Autodesk Fusion 360 part; units mm, degrees
note: some values were not read from the file. Set by a fixed rule: which face or edge a step refers to.
(part 2 of 2)
  line L1239 (389, 358.5) -> (389, 338.5)
  line L1240 (389, 338.5) -> (409, 338.5)
  line L1241 (409, 338.5) -> (409, 358.5)
  line L1242 (433, 358.5) -> (413, 358.5)
  line L1243 (413, 358.5) -> (413, 338.5)
  line L1244 (413, 338.5) -> (433, 338.5)
  line L1245 (433, 338.5) -> (433, 358.5)
  line L1246 (457, 358.5) -> (437, 358.5)
  line L1247 (437, 358.5) -> (437, 338.5)
  line L1248 (437, 338.5) -> (457, 338.5)
  line L1249 (457, 338.5) -> (457, 358.5)
  line L1250 (481, 358.5) -> (461, 358.5)
  line L1251 (461, 358.5) -> (461, 338.5)
  line L1252 (461, 338.5) -> (481, 338.5)
  line L1253 (481, 338.5) -> (481, 358.5)
  line L1254 (313, 382.5) -> (293, 382.5)
  line L1255 (293, 382.5) -> (293, 362.5)
  line L1256 (293, 362.5) -> (313, 362.5)
  line L1257 (313, 362.5) -> (313, 382.5)
  line L1258 (337, 382.5) -> (317, 382.5)
  line L1259 (317, 382.5) -> (317, 362.5)
  line L1260 (317, 362.5) -> (337, 362.5)
  line L1261 (337, 362.5) -> (337, 382.5)
  line L1262 (361, 382.5) -> (341, 382.5)
  line L1263 (341, 382.5) -> (341, 362.5)
  line L1264 (341, 362.5) -> (361, 362.5)
  line L1265 (361, 362.5) -> (361, 382.5)
  line L1266 (385, 382.5) -> (365, 382.5)
  line L1267 (365, 382.5) -> (365, 362.5)
  line L1268 (365, 362.5) -> (385, 362.5)
  line L1269 (385, 362.5) -> (385, 382.5)
  line L1270 (409, 382.5) -> (389, 382.5)
  line L1271 (389, 382.5) -> (389, 362.5)
  line L1272 (389, 362.5) -> (409, 362.5)
  line L1273 (409, 362.5) -> (409, 382.5)
  line L1274 (433, 382.5) -> (413, 382.5)
  line L1275 (413, 382.5) -> (413, 362.5)
  line L1276 (413, 362.5) -> (433, 362.5)
  line L1277 (433, 362.5) -> (433, 382.5)
  line L1278 (457, 382.5) -> (437, 382.5)
  line L1279 (437, 382.5) -> (437, 362.5)
  line L1280 (437, 362.5) -> (457, 362.5)
  line L1281 (457, 362.5) -> (457, 382.5)
  line L1282 (481, 382.5) -> (461, 382.5)
  line L1283 (461, 382.5) -> (461, 362.5)
  line L1284 (461, 362.5) -> (481, 362.5)
  line L1285 (481, 362.5) -> (481, 382.5)
  dimension "d46" = 486
  dimension "d47" = 385
  dimension "d50" = 5
  dimension "d51" = 2.5
  dimension "d52" = 20
  dimension "d53" = 20
  dimension "d56" = 24
  dimension "d57" = 24
  constraint horizontal L0
  constraint vertical L1
  constraint horizontal L2
  constraint vertical L3
  constraint coincident L0.start L3.end
  constraint coincident L3 L4.end
  constraint perpendicular L3 L4
  constraint coincident L0 L5.end
  constraint perpendicular L0 L5
  constraint horizontal L6
  constraint vertical L7
  constraint horizontal L8
  constraint vertical L9
  measures "d46" distance of L0.start L0.end
  measures "d47" distance of L0.start L2.end
  measures "d50" distance of L4.start L4.end
  measures "d51" distance of L4.start L5.end
  measures "d52" distance of L4.start L6.end
  measures "d53" distance of L4.start L8.end
extrude "Extrude2" add sketch "Sketch4" along normal blind 3 makes body 1
box "BoxPrimitive1" add length 24 width 22 height 51 placed x (0, 1, 0) y (-1, 0, 0) z (0, 0, 1) at (29, 369, 3) separate body makes body 2
extrude "Extrude3" cut 1 faces at (14.3333, 377, 3) along direction (0, 0, 1) blind 1 on bodies 2 bodies 2
extrude "Extrude4" cut 1 faces at (21.6667, 393, 20.6667) along direction (0, -1, 0) blind 2 on bodies 2 bodies 2
box "BoxPrimitive2" add length 19 width 19 height 4 placed x (0, 1, 0) y (1, 0, 0) z (0, 0, -1) at (8.5, 370.5, 4) bodies 2
shell "Shell1" thickness 2 removed faces 1 at (21.6667, 376.3333, 54) on bodies 2
copy_body "CopyPasteBodies1" bodies 2 makes body 3
move_body "Move1" bodies 3 to x (1, 0, 0) y (0, 1, 0) z (0, 0, 1) at (0, -24, 0)
copy_body "CopyPasteBodies2" bodies 3 2 makes body 4 makes body 5
move_body "Move2" bodies 4 5 to x (1, 0, 0) y (0, 1, 0) z (0, 0, 1) at (24, 0, 0)
copy_body "CopyPasteBodies3" bodies 3 2 4 5 makes body 6 makes body 7 makes body 8 makes body 9
move_body "Move3" bodies 6 7 8 9 to x (1, 0, 0) y (0, 1, 0) z (0, 0, 1) at (0, -72, 0)
box "BoxPrimitive3" add length 46 width 46 height -50 placed x (0, -1, 0) y (1, 0, 0) z (0, 0, 1) at (7, 319, 54) bodies 6 7 8 9
extrude "Extrude5" add 4 faces at (21.1667, 280.8333, 0) (38.8333, 280.8333, 0) (21.1667, 304.8333, 0) (38.8333, 304.8333, 0) along direction (0, 0, 1) blind 5 on bodies 6 bodies 6
shell "Shell2" thickness 2 removed faces 1 at (37.6667, 280.3333, 54) on bodies 6
extrude "Extrude6" add 4 faces at (44.5, 305.5, 2) (20.5, 305.5, 2) (44.5, 281.5, 2) (20.5, 281.5, 2) along direction (0, 0, 1) blind 4 on bodies 6 bodies 6
extrude "Extrude7" add 4 faces at (44.5, 353.5, 2) (44.5, 377.5, 2) (20.5, 377.5, 2) (20.5, 353.5, 2) along direction (0, 0, 1) blind 4 on bodies 2 3 4 5 bodies 4 2 3 5
copy_body "CopyPasteBodies4" bodies 6 makes body 10
move_body "Move4" bodies 10 to x (1, 0, 0) y (0, 1, 0) z (0, 0, 1) at (0, -72, 0)
copy_body "CopyPasteBodies5" bodies 10 makes body 11
move_body "Move5" bodies 11 to x (1, 0, 0) y (0, 1, 0) z (0, 0, 1) at (48, 0, 0)
box "BoxPrimitive4" add length 46 width 94 height -50 placed x (0, 1, 0) y (-1, 0, 0) z (0, 0, 1) at (101, 201, 54) bodies 10 11
shell "Shell3" thickness 2 removed faces 1 at (70.3333, 223.6667, 54) on bodies 10
extrude "Extrude8" add 8 faces at (68.5, 233.5, 2) (44.5, 233.5, 2) (20.5, 233.5, 2) (20.5, 209.5, 2) (44.5, 209.5, 2) (68.5, 209.5, 2) (92.5, 209.5, 2) (92.5, 233.5, 2) along direction (0, 0, 1) blind 4 on bodies 10 bodies 10
copy_body "CopyPasteBodies6" bodies 10 makes body 12
move_body "Move6" bodies 12 to x (1, 0, 0) y (0, 1, 0) z (0, 0, 1) at (0, -72, 0)
copy_body "CopyPasteBodies7" bodies 12 makes body 13
move_body "Move7" bodies 13 to x (1, 0, 0) y (0, 1, 0) z (0, 0, 1) at (0, -48, 0)
box "BoxPrimitive5" add length 94 width 94 height -50 placed x (0, 1, 0) y (-1, 0, 0) z (0, 0, 1) at (101, 81, 54) bodies 12 13
shell "Shell4" thickness 2 removed faces 1 at (54.3333, 113, 54) on bodies 12
extrude "Extrude9" add 16 faces at (20.5, 89.5, 2) (20.5, 113.5, 2) (44.5, 89.5, 2) (44.5, 113.5, 2) (68.5, 113.5, 2) (68.5, 89.5, 2) (92.5, 89.5, 2) (92.5, 113.5, 2) (92.5, 137.5, 2) (68.5, 137.5, 2) (44.5, 137.5, 2) (20.5, 137.5, 2) (20.5, 161.5, 2) (44.5, 161.5, 2) (68.5, 161.5, 2) (92.5, 161.5, 2) along direction (0, 0, 1) blind 4 on bodies 12 bodies 12
copy_body "CopyPasteBodies8" bodies 6 makes body 14
move_body "Move8" bodies 14 to x (1, 0, 0) y (0, 1, 0) z (0, 0, 1) at (72, 0, 0)
copy_body "CopyPasteBodies9" bodies 14 makes body 15
move_body "Move9" bodies 15 to x (1, 0, 0) y (0, 1, 0) z (0, 0, 1) at (0, 24, 0)
copy_body "CopyPasteBodies10" bodies 15 14 makes body 16 makes body 17
move_body "Move10" bodies 16 17 to x (1, 0, 0) y (0, 1, 0) z (0, 0, 1) at (24, 0, 0)
box "BoxPrimitive6" add length 70 width 70 height -50 placed x (0, -1, 0) y (1, 0, 0) z (0, 0, 1) at (79, 343, 54) bodies 14 15 16 17
shell "Shell5" thickness 2 removed faces 1 at (102.3333, 328.3333, 54) on bodies 14
extrude "Extrude10" add 9 faces at (140.5, 305.5, 2) (140.5, 329.5, 2) (140.5, 281.5, 2) (116.5, 281.5, 2) (116.5, 305.5, 2) (116.5, 329.5, 2) (92.5, 329.5, 2) (92.5, 281.5, 2) (92.5, 305.5, 2) along direction (0, 0, 1) blind 4 on bodies 14 bodies 14
copy_body "CopyPasteBodies11" bodies 5 2 makes body 18 makes body 19
move_body "Move11" bodies 18 19 to x (1, 0, 0) y (0, 1, 0) z (0, 0, 1) at (168, -24, 0)
copy_body "CopyPasteBodies12" bodies 19 18 makes body 20 makes body 21
move_body "Move12" bodies 20 21 to x (1, 0, 0) y (0, 1, 0) z (0, 0, 1) at (48, 0, 0)
box "BoxPrimitive7" add length 22 width 94 height -50 placed x (0, -1, 0) y (1, 0, 0) z (0, 0, 1) at (175, 367, 54) bodies 18 19 20 21
shell "Shell6" thickness 2 removed faces 1 at (237.6667, 352.3333, 54) on bodies 18
extrude "Extrude11" add 4 faces at (188.5, 353.5, 2) (212.5, 353.5, 2) (236.5, 353.5, 2) (260.5, 353.5, 2) along direction (0, 0, 1) blind 4 on bodies 18 bodies 18
move_body "Move13" bodies 2 18 3 5 14 10 4 12 6 to x (1, 0, 0) y (0, 1, 0) z (0, 0, 1) at (-3, -8, 0)
copy_body "CopyPasteBodies13" bodies 12 makes body 22
move_body "Move14" bodies 22 to x (1, 0, 0) y (0, 1, 0) z (0, 0, 1) at (120, 0, 0)
copy_body "CopyPasteBodies14" bodies 22 makes body 23
move_body "Move15" bodies 23 to x (1, 0, 0) y (0, 1, 0) z (0, 0, 1) at (0, -24, 0)
copy_body "CopyPasteBodies15" bodies 22 23 makes body 24 makes body 25
move_body "Move16" bodies 24 25 to x (1, 0, 0) y (0, 1, 0) z (0, 0, 1) at (24, 0, 0)
box "BoxPrimitive8" add length 118 width 118 height -50 placed x (0, -1, 0) y (1, 0, 0) z (0, 0, 1) at (124, 167, 54) bodies 22 23 24 25
shell "Shell7" thickness 2 removed faces 1 at (195.3333, 104.3333, 54) on bodies 22
extrude "Extrude12" add 25 faces at (137.5, 57.5, 2) (137.5, 81.5, 2) (137.5, 105.5, 2) (137.5, 129.5, 2) (137.5, 153.5, 2) (161.5, 153.5, 2) (161.5, 129.5, 2) (161.5, 105.5, 2) (161.5, 81.5, 2) (161.5, 57.5, 2) (185.5, 57.5, 2) (185.5, 81.5, 2) (185.5, 129.5, 2) (185.5, 153.5, 2) (185.5, 105.5, 2) (209.5, 129.5, 2) (209.5, 105.5, 2) (209.5, 81.5, 2) (209.5, 57.5, 2) (233.5, 57.5, 2) (233.5, 81.5, 2) (233.5, 105.5, 2) (233.5, 129.5, 2) (233.5, 153.5, 2) (209.5, 153.5, 2) along direction (0, 0, 1) blind 4 on bodies 22 bodies 22
copy_body "CopyPasteBodies16" bodies 10 makes body 26
move_body "Move17" bodies 26 to x (1, 0, 0) y (0, 1, 0) z (0, 0, 1) at (288, 0, 0)
move_body "Move18" bodies 6 to x (1, 0, 0) y (0, 1, 0) z (0, 0, 1) at (384, -72, 0)
copy_body "CopyPasteBodies17" bodies 6 makes body 27
move_body "Move19" bodies 27 to x (1, 0, 0) y (0, 1, 0) z (0, 0, 1) at (0, 0, 0)
move_body "Move20" bodies 6 to x (1, 0, 0) y (0, 1, 0) z (0, 0, 1) at (0, -120, 0)
copy_body "CopyPasteBodies18" bodies 26 makes body 28
move_body "Move21" bodies 28 to x (0, 1, 0) y (-1, 0, 0) z (0, 0, 1) at (627, -51, 0)
box "BoxPrimitive9" add length 142 width 46 height -50 placed x (0, -1, 0) y (1, 0, 0) z (0, 0, 1) at (388, 335, 54) bodies 27 28
box "BoxPrimitive10" add length 46 width 142 height -50 placed x (0, 1, 0) y (-1, 0, 0) z (0, 0, 1) at (434, 193, 54) bodies 26 27
shell "Shell8" thickness 2 removed faces 1 at (411.3333, 304.3333, 54) on bodies 26
extrude "Extrude13" add 20 faces at (401.5, 326.5, 2) (425.5, 326.5, 2) (425.5, 302.5, 2) (401.5, 302.5, 2) (425.5, 278.5, 2) (401.5, 278.5, 2) (425.5, 249.5, 2) (401.5, 249.5, 2) (401.5, 225.5, 2) (425.5, 225.5, 2) (425.5, 201.5, 2) (401.5, 201.5, 2) (377.5, 201.5, 2) (353.5, 201.5, 2) (329.5, 201.5, 2) (305.5, 201.5, 2) (305.5, 225.5, 2) (329.5, 225.5, 2) (353.5, 225.5, 2) (377.5, 225.5, 2) along direction (0, 0, 1) blind 4 on bodies 26 bodies 26
equation "Width = widthactual - 1" comment "Width"
equation "WidthMM = Width * 1 mm" comment "Width in MM"
equation "Length = lengthactual - 1" comment "Length"
equation "LengthMM = Length * 1 mm" comment "Length in MM"
equation "Peg = 20" comment "Peg"
equation "PegMM = Peg * 1 mm" comment "Peg in MM"
equation "Wall = Peg + WallSize" comment "Wall"
equation "WallMM = Wall * 1 mm" comment "Wall in MM"
equation "PegWidth = floor(Width / Wall)"
equation "PegLength = floor(Length / Wall)"
equation "LipW = ( ( Width - ( ( PegWidth * Wall ) - WallSize ) ) / 2 ) * 1 mm"
equation "LipL = ( ( Length - ( ( PegLength * Wall ) - WallSize ) ) / 2 ) * 1 mm"
equation "d46 = WidthMM"
equation "d47 = LengthMM"
equation "d50 = LipW"
equation "d51 = LipL"
equation "d52 = PegMM"
equation "d53 = PegMM"
equation "d54 = PegWidth"
equation "d55 = PegLength"
equation "d56 = WallMM"
equation "d57 = WallMM"
equation "WallSize = 4" comment "WALL SIZE HERE"
equation "d64 = BucketHeight"
equation "d79 = bucketheightneg"
equation "d91 = bucketheightneg"
equation "d99 = bucketheightneg"
equation "d107 = bucketheightneg"
equation "d115 = bucketheightneg"
equation "widthactual = 487"
equation "lengthactual = 386"
equation "d125 = bucketheightneg"
equation "d133 = bucketheightneg"
equation "d138 = bucketheightneg"
equation "BucketHeight = bucketheightactual + 1 mm"
equation "bucketheightactual = 50 mm"
equation "bucketheightneg = -bucketheightactual"
